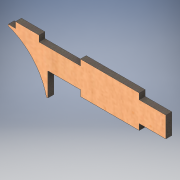
# Autodesk Inventor part: spacer
Saved by Autodesk Inventor 2019 (Build 230136000, 136)
## iProperties
Created: 2020-12-06
Part Number: spacer
Material: Дерево (береза)
Document SubType Name: Modeling
Designer: Professional
Density: 0.55 g/cm^3
Appearance: Береза — натуральный — полированный
Author: Professional
Autodesk Inventor part; units mm, degrees
ref_plane "YZ Plane" through (0, 0, 0) normal (1, 0, 0) x (0, 1, 0)
ref_plane "XZ Plane" through (0, 0, 0) normal (0, 1, 0) x (-1, 0, 0)
ref_plane "XY Plane" through (0, 0, 0) normal (0, 0, 1) x (1, 0, 0)
sketch "Эскиз1" plane through (0, 0, 0) normal (0, 0, 1) x (1, 0, 0)
  line L0 (0, 0) -> (38, 0)
  line L1 (-42, -7) -> (-20, -7)
  line L2 (-20, -7) -> (-20, -11)
  line L3 (-20, -11) -> (0, -11)
  line L4 (0, -11) -> (0, 0)
  line L5 (-42, 7) -> (-20, 7)
  line L6 (-20, 7) -> (-20, 11)
  line L7 (-20, 11) -> (0, 11)
  line L8 (0, 11) -> (0, 0)
  line L9 (20, -7) -> (20, -11)
  line L10 (20, -11) -> (0, -11)
  line L11 (20, 7) -> (20, 11)
  line L12 (20, 11) -> (0, 11)
  line L13 (-42, -7) -> (-42, -22.9118)
  line L14 (-42, -22.9118) -> (-43, -22.9118)
  arc A0 (-43, -22.9118) -> (-68.9172, 6) centre (-82, -31.8) ccw
  line L15 (-68.9172, 7) -> (-64, 7)
  line L16 (-64, 7) -> (-64, 11)
  line L17 (-64, 11) -> (-48, 11)
  line L18 (-48, 11) -> (-48, 7)
  line L19 (-48, 7) -> (-42, 7)
  line L20 (-68.9172, 6) -> (-68.9172, 7)
  line L21 (20, -7) -> (38, -7)
  line L22 (38, -7) -> (38, 7)
  line L23 (38, 7) -> (20, 7)
  dimension "d1" = 14
  dimension "d2" = 4
  dimension "d3" = 40
  dimension "d7" = 40
  dimension "d8" = 38.8
  dimension "d9" = 40
  dimension "d10" = 1
  dimension "d11" = 16
  dimension "d12" = 6
  dimension "d13" = 42
  dimension "d15" = 38
  constraints: 48 end point, 8 perpendicular, 8 symmetric about line, 3 horizontal, 3 vertical, 2 equal length, 2 point on circle, 1 centre point, 1 collinear, 1 midpoint, 1 point on line
  measures "d1" diameter of L1 L0
  measures "d2" distance of L1.end L2.end
  measures "d3" diameter of L2 L4
  measures "d7" radius of A0
  measures "d8" distance from line of A0.centre L15
  measures "d9" distance from line of L13 A0.centre
  measures "d10" distance of L13.end L14.end
  measures "d11" distance between parallel lines of L16 L18
  measures "d12" distance between parallel lines of L13 L18
  measures "d13" distance from line of L13 L7.end
  measures "d15" distance from line of L22 L3.end
extrude "Выдавливание1" add sketch "Эскиз1" along normal blind 4
